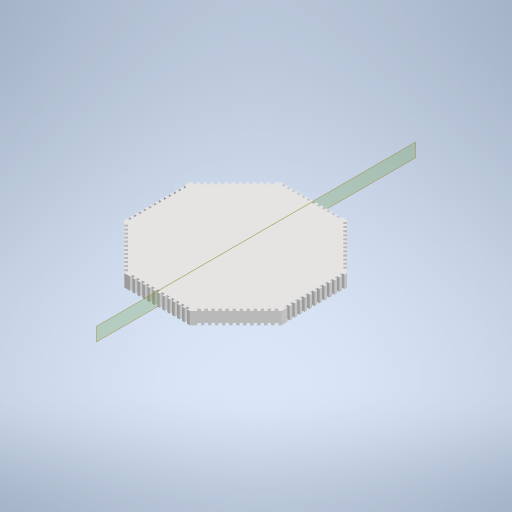
# Autodesk Inventor part: pla
Saved by Autodesk Inventor 2023 (Build 270158000, 158)
## iProperties
Created: 2023-04-19
Part Number: pla
Material: 일반
Document SubType Name: Modeling
Designer: didtk
Density: 1 g/cm^3
Appearance: 기본값
Author: didtk
Autodesk Inventor part; units mm, degrees
(part 1 of 2)
ref_plane "YZ Plane" through (0, 0, 0) normal (1, 0, 0) x (0, 1, 0)
ref_plane "XZ Plane" through (0, 0, 0) normal (0, 1, 0) x (-1, 0, 0)
ref_plane "XY Plane" through (0, 0, 0) normal (0, 0, 1) x (1, 0, 0)
sketch "스케치1" plane through (0, 0, 0) normal (0, 1, 0) x (-1, 0, 0)
  line L0 (26.6174, 64.26) -> (27.3245, 63.5529)
  line L1 (27.3245, 63.5529) -> (26.6174, 62.8458)
  line L2 (27.3245, 62.1387) -> (26.6174, 62.8458)
  line L3 (28.0316, 62.8458) -> (27.3245, 62.1387)
  line L4 (28.0316, 62.8458) -> (28.7387, 62.1387)
  line L5 (28.7387, 62.1387) -> (28.0316, 61.4316)
  line L6 (28.7387, 60.7245) -> (28.0316, 61.4316)
  line L7 (29.4458, 61.4316) -> (28.7387, 60.7245)
  line L8 (29.4458, 61.4316) -> (30.1529, 60.7245)
  line L9 (30.1529, 60.7245) -> (29.4458, 60.0174)
  line L10 (30.1529, 59.3103) -> (29.4458, 60.0174)
  line L11 (30.86, 60.0174) -> (30.1529, 59.3103)
  line L12 (30.86, 60.0174) -> (31.5671, 59.3103)
  line L13 (31.5671, 59.3103) -> (30.86, 58.6032)
  line L14 (31.5671, 57.896) -> (30.86, 58.6032)
  line L15 (32.2742, 58.6032) -> (31.5671, 57.896)
  line L16 (32.2742, 58.6032) -> (32.9813, 57.896)
  line L17 (32.9813, 57.896) -> (32.2742, 57.1889)
  line L18 (32.9813, 56.4818) -> (32.2742, 57.1889)
  line L19 (33.6884, 57.1889) -> (32.9813, 56.4818)
  line L20 (33.6884, 57.1889) -> (34.3955, 56.4818)
  line L21 (34.3955, 56.4818) -> (33.6884, 55.7747)
  line L22 (34.3955, 55.0676) -> (33.6884, 55.7747)
  line L23 (35.1026, 55.7747) -> (34.3955, 55.0676)
  line L24 (35.1026, 55.7747) -> (35.8098, 55.0676)
  line L25 (35.8098, 55.0676) -> (35.1026, 54.3605)
  line L26 (35.8098, 53.6534) -> (35.1026, 54.3605)
  line L27 (36.5169, 54.3605) -> (35.8098, 53.6534)
  line L28 (36.5169, 54.3605) -> (37.224, 53.6534)
  line L29 (37.224, 53.6534) -> (36.5169, 52.9463)
  line L30 (37.224, 52.2392) -> (36.5169, 52.9463)
  line L31 (37.9311, 52.9463) -> (37.224, 52.2392)
  line L32 (37.9311, 52.9463) -> (38.6382, 52.2392)
  line L33 (38.6382, 52.2392) -> (37.9311, 51.5321)
  line L34 (38.6382, 50.825) -> (37.9311, 51.5321)
  line L35 (39.3453, 51.5321) -> (38.6382, 50.825)
  line L36 (39.3453, 51.5321) -> (40.0524, 50.825)
  line L37 (40.0524, 50.825) -> (39.3453, 50.1179)
  line L38 (40.0524, 49.4108) -> (39.3453, 50.1179)
  line L39 (40.7595, 50.1179) -> (40.0524, 49.4108)
  line L40 (40.7595, 50.1179) -> (41.4666, 49.4108)
  line L41 (41.4666, 49.4108) -> (40.7595, 48.7037)
  line L42 (41.4666, 47.9965) -> (40.7595, 48.7037)
  line L43 (42.1737, 48.7037) -> (41.4666, 47.9965)
  line L44 (42.1737, 48.7037) -> (42.8808, 47.9965)
  line L45 (42.8808, 47.9965) -> (42.1737, 47.2894)
  line L46 (42.8808, 46.5823) -> (42.1737, 47.2894)
  line L47 (43.5879, 47.2894) -> (42.8808, 46.5823)
  line L48 (43.5879, 47.2894) -> (45.1681, 45.7092)
  line L49 (45.1681, 45.7092) -> (45.1681, 44.7092)
  line L50 (45.1681, 44.7092) -> (44.1681, 44.7092)
  line L51 (44.1681, 43.7092) -> (44.1681, 44.7092)
  line L52 (45.1681, 43.7092) -> (44.1681, 43.7092)
  line L53 (45.1681, 43.7092) -> (45.1681, 42.7092)
  line L54 (45.1681, 42.7092) -> (44.1681, 42.7092)
  line L55 (44.1681, 41.7092) -> (44.1681, 42.7092)
  line L56 (45.1681, 41.7092) -> (44.1681, 41.7092)
  line L57 (45.1681, 41.7092) -> (45.1681, 40.7092)
  line L58 (45.1681, 40.7092) -> (44.1681, 40.7092)
  line L59 (44.1681, 39.7092) -> (44.1681, 40.7092)
  line L60 (45.1681, 39.7092) -> (44.1681, 39.7092)
  line L61 (45.1681, 39.7092) -> (45.1681, 38.7092)
  line L62 (45.1681, 38.7092) -> (44.1681, 38.7092)
  line L63 (44.1681, 37.7092) -> (44.1681, 38.7092)
  line L64 (45.1681, 37.7092) -> (44.1681, 37.7092)
  line L65 (45.1681, 37.7092) -> (45.1681, 36.7092)
  line L66 (45.1681, 36.7092) -> (44.1681, 36.7092)
  line L67 (44.1681, 35.7092) -> (44.1681, 36.7092)
  line L68 (45.1681, 35.7092) -> (44.1681, 35.7092)
  line L69 (45.1681, 35.7092) -> (45.1681, 34.7092)
  line L70 (45.1681, 34.7092) -> (44.1681, 34.7092)
  line L71 (44.1681, 33.7092) -> (44.1681, 34.7092)
  line L72 (45.1681, 33.7092) -> (44.1681, 33.7092)
  line L73 (45.1681, 33.7092) -> (45.1681, 32.7092)
  line L74 (45.1681, 32.7092) -> (44.1681, 32.7092)
  line L75 (44.1681, 31.7092) -> (44.1681, 32.7092)
  line L76 (45.1681, 31.7092) -> (44.1681, 31.7092)
  line L77 (45.1681, 31.7092) -> (45.1681, 30.7092)
  line L78 (45.1681, 30.7092) -> (44.1681, 30.7092)
  line L79 (44.1681, 29.7092) -> (44.1681, 30.7092)
  line L80 (45.1681, 29.7092) -> (44.1681, 29.7092)
  line L81 (45.1681, 29.7092) -> (45.1681, 28.7092)
  line L82 (45.1681, 28.7092) -> (44.1681, 28.7092)
  line L83 (44.1681, 27.7092) -> (44.1681, 28.7092)
  line L84 (45.1681, 27.7092) -> (44.1681, 27.7092)
  line L85 (45.1681, 27.7092) -> (45.1681, 26.7092)
  line L86 (45.1681, 26.7092) -> (44.1681, 26.7092)
  line L87 (44.1681, 25.7092) -> (44.1681, 26.7092)
  line L88 (45.1681, 25.7092) -> (44.1681, 25.7092)
  line L89 (45.1681, 25.7092) -> (45.1681, 24.7092)
  line L90 (45.1681, 24.7092) -> (44.1681, 24.7092)
  line L91 (44.1681, 23.7092) -> (44.1681, 24.7092)
  line L92 (45.1681, 23.7092) -> (44.1681, 23.7092)
  line L93 (45.1681, 23.7092) -> (45.1681, 22.7092)
  line L94 (45.1681, 22.7092) -> (44.1681, 22.7092)
  line L95 (44.1681, 21.7092) -> (44.1681, 22.7092)
  line L96 (45.1681, 21.7092) -> (44.1681, 21.7092)
  line L97 (45.1681, 21.7092) -> (45.1681, 19.4745)
  line L98 (45.1681, 19.4745) -> (44.461, 18.7674)
  line L99 (44.461, 18.7674) -> (43.7539, 19.4745)
  line L100 (43.0468, 18.7674) -> (43.7539, 19.4745)
  line L101 (43.7539, 18.0603) -> (43.0468, 18.7674)
  line L102 (43.7539, 18.0603) -> (43.0468, 17.3532)
  line L103 (43.0468, 17.3532) -> (42.3397, 18.0603)
  line L104 (41.6326, 17.3532) -> (42.3397, 18.0603)
  line L105 (42.3397, 16.6461) -> (41.6326, 17.3532)
  line L106 (42.3397, 16.6461) -> (41.6326, 15.939)
  line L107 (41.6326, 15.939) -> (40.9255, 16.6461)
  line L108 (40.2184, 15.939) -> (40.9255, 16.6461)
  line L109 (40.9255, 15.2319) -> (40.2184, 15.939)
  line L110 (40.9255, 15.2319) -> (40.2184, 14.5248)
  line L111 (40.2184, 14.5248) -> (39.5113, 15.2319)
  line L112 (38.8042, 14.5248) -> (39.5113, 15.2319)
  line L113 (39.5113, 13.8177) -> (38.8042, 14.5248)
  line L114 (39.5113, 13.8177) -> (38.8042, 13.1106)
  line L115 (38.8042, 13.1106) -> (38.0971, 13.8177)
  line L116 (37.3899, 13.1106) -> (38.0971, 13.8177)
  line L117 (38.0971, 12.4034) -> (37.3899, 13.1106)
  line L118 (38.0971, 12.4034) -> (37.3899, 11.6963)
  line L119 (37.3899, 11.6963) -> (36.6828, 12.4034)
  line L120 (35.9757, 11.6963) -> (36.6828, 12.4034)
  line L121 (36.6828, 10.9892) -> (35.9757, 11.6963)
  line L122 (36.6828, 10.9892) -> (35.9757, 10.2821)
  line L123 (35.9757, 10.2821) -> (35.2686, 10.9892)
  line L124 (34.5615, 10.2821) -> (35.2686, 10.9892)
  line L125 (35.2686, 9.575) -> (34.5615, 10.2821)
  line L126 (35.2686, 9.575) -> (34.5615, 8.8679)
  line L127 (34.5615, 8.8679) -> (33.8544, 9.575)
  line L128 (33.1473, 8.8679) -> (33.8544, 9.575)
  line L129 (33.8544, 8.1608) -> (33.1473, 8.8679)
  line L130 (33.8544, 8.1608) -> (33.1473, 7.4537)
  line L131 (33.1473, 7.4537) -> (32.4402, 8.1608)
  line L132 (31.7331, 7.4537) -> (32.4402, 8.1608)
  line L133 (32.4402, 6.7466) -> (31.7331, 7.4537)
  line L134 (32.4402, 6.7466) -> (31.7331, 6.0395)
  line L135 (31.7331, 6.0395) -> (31.026, 6.7466)
  line L136 (30.3189, 6.0395) -> (31.026, 6.7466)
  line L137 (31.026, 5.3324) -> (30.3189, 6.0395)
  line L138 (31.026, 5.3324) -> (30.3189, 4.6253)
  line L139 (30.3189, 4.6253) -> (29.6118, 5.3324)
  line L140 (28.9047, 4.6253) -> (29.6118, 5.3324)
  line L141 (29.6118, 3.9182) -> (28.9047, 4.6253)
  line L142 (29.6118, 3.9182) -> (28.9047, 3.2111)
  line L143 (28.9047, 3.2111) -> (28.1976, 3.9182)
  line L144 (27.4905, 3.2111) -> (28.1976, 3.9182)
  line L145 (28.1976, 2.504) -> (27.4905, 3.2111)
  line L146 (28.1976, 2.504) -> (26.6174, 0.9238)
  line L147 (26.6174, 0.9238) -> (25.6174, 0.9238)
  line L148 (25.6174, 0.9238) -> (25.6174, 1.9238)
  line L149 (24.6174, 1.9238) -> (25.6174, 1.9238)
  line L150 (24.6174, 0.9238) -> (24.6174, 1.9238)
  line L151 (24.6174, 0.9238) -> (23.6174, 0.9238)
  line L152 (23.6174, 0.9238) -> (23.6174, 1.9238)
  line L153 (22.6174, 1.9238) -> (23.6174, 1.9238)
  line L154 (22.6174, 0.9238) -> (22.6174, 1.9238)
  line L155 (22.6174, 0.9238) -> (21.6174, 0.9238)
  line L156 (21.6174, 0.9238) -> (21.6174, 1.9238)
  line L157 (20.6174, 1.9238) -> (21.6174, 1.9238)
  line L158 (20.6174, 0.9238) -> (20.6174, 1.9238)
  line L159 (20.6174, 0.9238) -> (19.6174, 0.9238)
  line L160 (19.6174, 0.9238) -> (19.6174, 1.9238)
  line L161 (18.6174, 1.9238) -> (19.6174, 1.9238)
  line L162 (18.6174, 0.9238) -> (18.6174, 1.9238)
  line L163 (18.6174, 0.9238) -> (17.6174, 0.9238)
  line L164 (17.6174, 0.9238) -> (17.6174, 1.9238)
  line L165 (16.6174, 1.9238) -> (17.6174, 1.9238)
  line L166 (16.6174, 0.9238) -> (16.6174, 1.9238)
  line L167 (16.6174, 0.9238) -> (15.6174, 0.9238)
  line L168 (15.6174, 0.9238) -> (15.6174, 1.9238)
  line L169 (14.6174, 1.9238) -> (15.6174, 1.9238)
  line L170 (14.6174, 0.9238) -> (14.6174, 1.9238)
  line L171 (14.6174, 0.9238) -> (13.6174, 0.9238)
  line L172 (13.6174, 0.9238) -> (13.6174, 1.9238)
  line L173 (12.6174, 1.9238) -> (13.6174, 1.9238)
  line L174 (12.6174, 0.9238) -> (12.6174, 1.9238)
  line L175 (12.6174, 0.9238) -> (11.6174, 0.9238)
  line L176 (11.6174, 0.9238) -> (11.6174, 1.9238)
  line L177 (10.6174, 1.9238) -> (11.6174, 1.9238)
  line L178 (10.6174, 0.9238) -> (10.6174, 1.9238)
  line L179 (10.6174, 0.9238) -> (9.6174, 0.9238)
  line L180 (9.6174, 0.9238) -> (9.6174, 1.9238)
  line L181 (8.6174, 1.9238) -> (9.6174, 1.9238)
  line L182 (8.6174, 0.9238) -> (8.6174, 1.9238)
  line L183 (8.6174, 0.9238) -> (7.6174, 0.9238)
  line L184 (7.6174, 0.9238) -> (7.6174, 1.9238)
  line L185 (6.6174, 1.9238) -> (7.6174, 1.9238)
  line L186 (6.6174, 0.9238) -> (6.6174, 1.9238)
  line L187 (6.6174, 0.9238) -> (5.6174, 0.9238)
  line L188 (5.6174, 0.9238) -> (5.6174, 1.9238)
  line L189 (4.6174, 1.9238) -> (5.6174, 1.9238)
  line L190 (4.6174, 0.9238) -> (4.6174, 1.9238)
  line L191 (4.6174, 0.9238) -> (3.6174, 0.9238)
  line L192 (3.6174, 0.9238) -> (3.6174, 1.9238)
  line L193 (2.6174, 1.9238) -> (3.6174, 1.9238)
  line L194 (2.6174, 0.9238) -> (2.6174, 1.9238)
  line L195 (2.6174, 0.9238) -> (0.3826, 0.9238)
  line L196 (0.3826, 0.9238) -> (-0.3245, 1.6309)
  line L197 (-0.3245, 1.6309) -> (0.3826, 2.338)
  line L198 (-0.3245, 3.0451) -> (0.3826, 2.338)
  line L199 (-1.0316, 2.338) -> (-0.3245, 3.0451)
  line L200 (-1.0316, 2.338) -> (-1.7387, 3.0451)
  line L201 (-1.7387, 3.0451) -> (-1.0316, 3.7522)
  line L202 (-1.7387, 4.4593) -> (-1.0316, 3.7522)
  line L203 (-2.4458, 3.7522) -> (-1.7387, 4.4593)
  line L204 (-2.4458, 3.7522) -> (-3.1529, 4.4593)
  line L205 (-3.1529, 4.4593) -> (-2.4458, 5.1664)
  line L206 (-3.1529, 5.8735) -> (-2.4458, 5.1664)
  line L207 (-3.86, 5.1664) -> (-3.1529, 5.8735)
  line L208 (-3.86, 5.1664) -> (-4.5671, 5.8735)
  line L209 (-4.5671, 5.8735) -> (-3.86, 6.5806)
  line L210 (-4.5671, 7.2877) -> (-3.86, 6.5806)
  line L211 (-5.2742, 6.5806) -> (-4.5671, 7.2877)
  line L212 (-5.2742, 6.5806) -> (-5.9813, 7.2877)
  line L213 (-5.9813, 7.2877) -> (-5.2742, 7.9948)
  line L214 (-5.9813, 8.7019) -> (-5.2742, 7.9948)
  line L215 (-6.6884, 7.9948) -> (-5.9813, 8.7019)
  line L216 (-6.6884, 7.9948) -> (-7.3955, 8.7019)
  line L217 (-7.3955, 8.7019) -> (-6.6884, 9.409)
  line L218 (-7.3955, 10.1161) -> (-6.6884, 9.409)
  line L219 (-8.1026, 9.409) -> (-7.3955, 10.1161)
  line L220 (-8.1026, 9.409) -> (-8.8098, 10.1161)
  line L221 (-8.8098, 10.1161) -> (-8.1026, 10.8233)
  line L222 (-8.8098, 11.5304) -> (-8.1026, 10.8233)
  line L223 (-9.5169, 10.8233) -> (-8.8098, 11.5304)
  line L224 (-9.5169, 10.8233) -> (-10.224, 11.5304)
  line L225 (-10.224, 11.5304) -> (-9.5169, 12.2375)
  line L226 (-10.224, 12.9446) -> (-9.5169, 12.2375)
  line L227 (-10.9311, 12.2375) -> (-10.224, 12.9446)
  line L228 (-10.9311, 12.2375) -> (-11.6382, 12.9446)
  line L229 (-11.6382, 12.9446) -> (-10.9311, 13.6517)
  line L230 (-11.6382, 14.3588) -> (-10.9311, 13.6517)
  line L231 (-12.3453, 13.6517) -> (-11.6382, 14.3588)
  line L232 (-12.3453, 13.6517) -> (-13.0524, 14.3588)
  line L233 (-13.0524, 14.3588) -> (-12.3453, 15.0659)
  line L234 (-13.0524, 15.773) -> (-12.3453, 15.0659)
  line L235 (-13.7595, 15.0659) -> (-13.0524, 15.773)
  line L236 (-13.7595, 15.0659) -> (-14.4666, 15.773)
  line L237 (-14.4666, 15.773) -> (-13.7595, 16.4801)
  line L238 (-14.4666, 17.1872) -> (-13.7595, 16.4801)
  line L239 (-15.1737, 16.4801) -> (-14.4666, 17.1872)
  line L240 (-15.1737, 16.4801) -> (-15.8808, 17.1872)
  line L241 (-15.8808, 17.1872) -> (-15.1737, 17.8943)
  line L242 (-15.8808, 18.6014) -> (-15.1737, 17.8943)
  line L243 (-16.5879, 17.8943) -> (-15.8808, 18.6014)
  line L244 (-16.5879, 17.8943) -> (-18.1681, 19.4745)
  line L245 (-18.1681, 19.4745) -> (-18.1681, 20.4745)
  line L246 (-18.1681, 20.4745) -> (-17.1681, 20.4745)
  line L247 (-17.1681, 21.4745) -> (-17.1681, 20.4745)
  line L248 (-18.1681, 21.4745) -> (-17.1681, 21.4745)
  line L249 (-18.1681, 21.4745) -> (-18.1681, 22.4745)
  line L250 (-18.1681, 22.4745) -> (-17.1681, 22.4745)
  line L251 (-17.1681, 23.4745) -> (-17.1681, 22.4745)
  line L252 (-18.1681, 23.4745) -> (-17.1681, 23.4745)
  line L253 (-18.1681, 23.4745) -> (-18.1681, 24.4745)
  line L254 (-18.1681, 24.4745) -> (-17.1681, 24.4745)
  line L255 (-17.1681, 25.4745) -> (-17.1681, 24.4745)
  line L256 (-18.1681, 25.4745) -> (-17.1681, 25.4745)
  line L257 (-18.1681, 25.4745) -> (-18.1681, 26.4745)
  line L258 (-18.1681, 26.4745) -> (-17.1681, 26.4745)
  line L259 (-17.1681, 27.4745) -> (-17.1681, 26.4745)
  line L260 (-18.1681, 27.4745) -> (-17.1681, 27.4745)
  line L261 (-18.1681, 27.4745) -> (-18.1681, 28.4745)
  line L262 (-18.1681, 28.4745) -> (-17.1681, 28.4745)
  line L263 (-17.1681, 29.4745) -> (-17.1681, 28.4745)
  line L264 (-18.1681, 29.4745) -> (-17.1681, 29.4745)
  line L265 (-18.1681, 29.4745) -> (-18.1681, 30.4745)
  line L266 (-18.1681, 30.4745) -> (-17.1681, 30.4745)
  line L267 (-17.1681, 31.4745) -> (-17.1681, 30.4745)
  line L268 (-18.1681, 31.4745) -> (-17.1681, 31.4745)
  line L269 (-18.1681, 31.4745) -> (-18.1681, 32.4745)
  line L270 (-18.1681, 32.4745) -> (-17.1681, 32.4745)
  line L271 (-17.1681, 33.4745) -> (-17.1681, 32.4745)
  line L272 (-18.1681, 33.4745) -> (-17.1681, 33.4745)
  line L273 (-18.1681, 33.4745) -> (-18.1681, 34.4745)
  line L274 (-18.1681, 34.4745) -> (-17.1681, 34.4745)
  line L275 (-17.1681, 35.4745) -> (-17.1681, 34.4745)
  line L276 (-18.1681, 35.4745) -> (-17.1681, 35.4745)
  line L277 (-18.1681, 35.4745) -> (-18.1681, 36.4745)
  line L278 (-18.1681, 36.4745) -> (-17.1681, 36.4745)
  line L279 (-17.1681, 37.4745) -> (-17.1681, 36.4745)
  line L280 (-18.1681, 37.4745) -> (-17.1681, 37.4745)
  line L281 (-18.1681, 37.4745) -> (-18.1681, 38.4745)
  line L282 (-18.1681, 38.4745) -> (-17.1681, 38.4745)
  line L283 (-17.1681, 39.4745) -> (-17.1681, 38.4745)
  line L284 (-18.1681, 39.4745) -> (-17.1681, 39.4745)
  line L285 (-18.1681, 39.4745) -> (-18.1681, 40.4745)
  line L286 (-18.1681, 40.4745) -> (-17.1681, 40.4745)
  line L287 (-17.1681, 41.4745) -> (-17.1681, 40.4745)
  line L288 (-18.1681, 41.4745) -> (-17.1681, 41.4745)
  line L289 (-18.1681, 41.4745) -> (-18.1681, 42.4745)
  line L290 (-18.1681, 42.4745) -> (-17.1681, 42.4745)
  line L291 (-17.1681, 43.4745) -> (-17.1681, 42.4745)
  line L292 (-18.1681, 43.4745) -> (-17.1681, 43.4745)
  line L293 (-18.1681, 43.4745) -> (-18.1681, 45.7092)
  line L294 (-18.1681, 45.7092) -> (-17.461, 46.4164)
  line L295 (-17.461, 46.4164) -> (-16.7539, 45.7092)
  line L296 (-16.0468, 46.4164) -> (-16.7539, 45.7092)
  line L297 (-16.7539, 47.1235) -> (-16.0468, 46.4164)
  line L298 (-16.7539, 47.1235) -> (-16.0468, 47.8306)
  line L299 (-16.0468, 47.8306) -> (-15.3397, 47.1235)
  line L300 (-14.6326, 47.8306) -> (-15.3397, 47.1235)
  line L301 (-15.3397, 48.5377) -> (-14.6326, 47.8306)
  line L302 (-15.3397, 48.5377) -> (-14.6326, 49.2448)
  line L303 (-14.6326, 49.2448) -> (-13.9255, 48.5377)
  line L304 (-13.2184, 49.2448) -> (-13.9255, 48.5377)
  line L305 (-13.9255, 49.9519) -> (-13.2184, 49.2448)
  line L306 (-13.9255, 49.9519) -> (-13.2184, 50.659)
  line L307 (-13.2184, 50.659) -> (-12.5113, 49.9519)
  line L308 (-11.8042, 50.659) -> (-12.5113, 49.9519)
  line L309 (-12.5113, 51.3661) -> (-11.8042, 50.659)
  line L310 (-12.5113, 51.3661) -> (-11.8042, 52.0732)
  line L311 (-11.8042, 52.0732) -> (-11.0971, 51.3661)
  line L312 (-10.3899, 52.0732) -> (-11.0971, 51.3661)
  line L313 (-11.0971, 52.7803) -> (-10.3899, 52.0732)
  line L314 (-11.0971, 52.7803) -> (-10.3899, 53.4874)
  line L315 (-10.3899, 53.4874) -> (-9.6828, 52.7803)
  line L316 (-8.9757, 53.4874) -> (-9.6828, 52.7803)
  line L317 (-9.6828, 54.1945) -> (-8.9757, 53.4874)
  line L318 (-9.6828, 54.1945) -> (-8.9757, 54.9016)
  line L319 (-8.9757, 54.9016) -> (-8.2686, 54.1945)
  line L320 (-7.5615, 54.9016) -> (-8.2686, 54.1945)
  line L321 (-8.2686, 55.6087) -> (-7.5615, 54.9016)
  line L322 (-8.2686, 55.6087) -> (-7.5615, 56.3159)
  line L323 (-7.5615, 56.3159) -> (-6.8544, 55.6087)
  line L324 (-6.1473, 56.3159) -> (-6.8544, 55.6087)
  line L325 (-6.8544, 57.023) -> (-6.1473, 56.3159)
  line L326 (-6.8544, 57.023) -> (-6.1473, 57.7301)
  line L327 (-6.1473, 57.7301) -> (-5.4402, 57.023)
  line L328 (-4.7331, 57.7301) -> (-5.4402, 57.023)
  line L329 (-5.4402, 58.4372) -> (-4.7331, 57.7301)
  line L330 (-5.4402, 58.4372) -> (-4.7331, 59.1443)
  line L331 (-4.7331, 59.1443) -> (-4.026, 58.4372)
  line L332 (-3.3189, 59.1443) -> (-4.026, 58.4372)
  line L333 (-4.026, 59.8514) -> (-3.3189, 59.1443)
  line L334 (-4.026, 59.8514) -> (-3.3189, 60.5585)
  line L335 (-3.3189, 60.5585) -> (-2.6118, 59.8514)
  line L336 (-1.9047, 60.5585) -> (-2.6118, 59.8514)
  line L337 (-2.6118, 61.2656) -> (-1.9047, 60.5585)
  line L338 (-2.6118, 61.2656) -> (-1.9047, 61.9727)
  line L339 (-1.9047, 61.9727) -> (-1.1976, 61.2656)
  line L340 (-0.4905, 61.9727) -> (-1.1976, 61.2656)
  line L341 (-1.1976, 62.6798) -> (-0.4905, 61.9727)
  line L342 (-1.1976, 62.6798) -> (0.3826, 64.26)
  line L343 (0.3826, 64.26) -> (1.3826, 64.26)
  line L344 (1.3826, 64.26) -> (1.3826, 63.26)
  line L345 (2.3826, 63.26) -> (1.3826, 63.26)
  line L346 (2.3826, 64.26) -> (2.3826, 63.26)
  line L347 (2.3826, 64.26) -> (3.3826, 64.26)
  line L348 (3.3826, 64.26) -> (3.3826, 63.26)
  line L349 (4.3826, 63.26) -> (3.3826, 63.26)
  line L350 (4.3826, 64.26) -> (4.3826, 63.26)
  line L351 (4.3826, 64.26) -> (5.3826, 64.26)
  line L352 (5.3826, 64.26) -> (5.3826, 63.26)
  line L353 (6.3826, 63.26) -> (5.3826, 63.26)
  line L354 (6.3826, 64.26) -> (6.3826, 63.26)
  line L355 (6.3826, 64.26) -> (7.3826, 64.26)
  line L356 (7.3826, 64.26) -> (7.3826, 63.26)
  line L357 (8.3826, 63.26) -> (7.3826, 63.26)
  line L358 (8.3826, 64.26) -> (8.3826, 63.26)
  line L359 (8.3826, 64.26) -> (9.3826, 64.26)
  line L360 (9.3826, 64.26) -> (9.3826, 63.26)
  line L361 (10.3826, 63.26) -> (9.3826, 63.26)
  line L362 (10.3826, 64.26) -> (10.3826, 63.26)
  line L363 (10.3826, 64.26) -> (11.3826, 64.26)
  line L364 (11.3826, 64.26) -> (11.3826, 63.26)
  line L365 (12.3826, 63.26) -> (11.3826, 63.26)
  line L366 (12.3826, 64.26) -> (12.3826, 63.26)
  line L367 (12.3826, 64.26) -> (13.3826, 64.26)
  line L368 (13.3826, 64.26) -> (13.3826, 63.26)
  line L369 (14.3826, 63.26) -> (13.3826, 63.26)
  line L370 (14.3826, 64.26) -> (14.3826, 63.26)
  line L371 (14.3826, 64.26) -> (15.3826, 64.26)
  line L372 (15.3826, 64.26) -> (15.3826, 63.26)
  line L373 (16.3826, 63.26) -> (15.3826, 63.26)
  line L374 (16.3826, 64.26) -> (16.3826, 63.26)
  line L375 (16.3826, 64.26) -> (17.3826, 64.26)
  line L376 (17.3826, 64.26) -> (17.3826, 63.26)
  line L377 (18.3826, 63.26) -> (17.3826, 63.26)
  line L378 (18.3826, 64.26) -> (18.3826, 63.26)
  line L379 (18.3826, 64.26) -> (19.3826, 64.26)
  line L380 (19.3826, 64.26) -> (19.3826, 63.26)
  line L381 (20.3826, 63.26) -> (19.3826, 63.26)
  line L382 (20.3826, 64.26) -> (20.3826, 63.26)
  line L383 (20.3826, 64.26) -> (21.3826, 64.26)
  line L384 (21.3826, 64.26) -> (21.3826, 63.26)
  line L385 (22.3826, 63.26) -> (21.3826, 63.26)
  line L386 (22.3826, 64.26) -> (22.3826, 63.26)
  line L387 (22.3826, 64.26) -> (23.3826, 64.26)
  line L388 (23.3826, 64.26) -> (23.3826, 63.26)
  line L389 (24.3826, 63.26) -> (23.3826, 63.26)
  line L390 (24.3826, 64.26) -> (24.3826, 63.26)
  line L391 (24.3826, 64.26) -> (26.6174, 64.26)
  line L392 (37.6421, 22.5919) -> (23.5, 8.4497)
  line L393 (23.5, 8.4497) -> (3.5, 8.4497)
  line L394 (3.5, 8.4497) -> (-10.6421, 22.5919)
  line L395 (-10.6421, 22.5919) -> (-10.6421, 42.5919)
  line L396 (-10.6421, 42.5919) -> (3.5, 56.734)
  line L397 (3.5, 56.734) -> (23.5, 56.734)
  line L398 (23.5, 56.734) -> (37.6421, 42.5919)
  line L399 (37.6421, 42.5919) -> (37.6421, 22.5919)
  point P0 (0, 0)
  point P1 (13.5, 32.5919)
  point P2 (13.5, 32.5919)
  dimension "d0" = 31.6681
  dimension "d1" = 31.6681
  dimension "d2" = 31.6681
  dimension "d3" = 31.6681
  dimension "d4" = 35.2772
  dimension "d5" = 20
  constraints: 800 end point, 1 coincident, 17 other
  measures "d0" distance from line of L371 point (13.5, 32.592)
  measures "d1" distance from line of L171 point (13.5, 32.592)
  measures "d2" distance from line of L73 point (13.5, 32.592)
  measures "d3" distance from line of L269 point (13.5, 32.592)
  measures "d4" distance of point (13.5, 32.592) point (0, 0)
  measures "d5" distance of L398.end L392.start
extrude "돌출1" add sketch "스케치1" along normal blind 5
sketch "스케치2" plane through (0, 0, 0) normal (0, 1, 0) x (-1, 0, 0)
  line L0 (29.4458, 60.0174) -> (30.1529, 60.7245) projected
  line L1 (30.1529, 60.7245) -> (29.4458, 61.4316) projected
  line L2 (29.4458, 61.4316) -> (28.7387, 60.7245) projected
  line L3 (28.7387, 60.7245) -> (28.0316, 61.4316) projected
  line L4 (28.0316, 61.4316) -> (28.7387, 62.1387) projected
  line L5 (28.7387, 62.1387) -> (28.0316, 62.8458) projected
  line L6 (28.0316, 62.8458) -> (27.3245, 62.1387) projected
  line L7 (27.3245, 62.1387) -> (26.6174, 62.8458) projected
  line L8 (26.6174, 62.8458) -> (27.3245, 63.5529) projected
  line L9 (27.3245, 63.5529) -> (26.6174, 64.26) projected
  line L10 (26.6174, 64.26) -> (24.3826, 64.26) projected
  line L11 (24.3826, 64.26) -> (24.3826, 63.26) projected
  line L12 (24.3826, 63.26) -> (23.3826, 63.26) projected
  line L13 (23.3826, 63.26) -> (23.3826, 64.26) projected
  line L14 (23.3826, 64.26) -> (22.3826, 64.26) projected
  line L15 (22.3826, 64.26) -> (22.3826, 63.26) projected
  line L16 (22.3826, 63.26) -> (21.3826, 63.26) projected
  line L17 (21.3826, 63.26) -> (21.3826, 64.26) projected
  line L18 (21.3826, 64.26) -> (20.3826, 64.26) projected
  line L19 (20.3826, 64.26) -> (20.3826, 63.26) projected
  line L20 (20.3826, 63.26) -> (19.3826, 63.26) projected
  line L21 (19.3826, 63.26) -> (19.3826, 64.26) projected
  line L22 (19.3826, 64.26) -> (18.3826, 64.26) projected
  line L23 (18.3826, 64.26) -> (18.3826, 63.26) projected
  line L24 (18.3826, 63.26) -> (17.3826, 63.26) projected
  line L25 (17.3826, 63.26) -> (17.3826, 64.26) projected
  line L26 (17.3826, 64.26) -> (16.3826, 64.26) projected
  line L27 (16.3826, 64.26) -> (16.3826, 63.26) projected
  line L28 (16.3826, 63.26) -> (15.3826, 63.26) projected
  line L29 (15.3826, 63.26) -> (15.3826, 64.26) projected
  line L30 (15.3826, 64.26) -> (14.3826, 64.26) projected
  line L31 (14.3826, 64.26) -> (14.3826, 63.26) projected
  line L32 (14.3826, 63.26) -> (13.3826, 63.26) projected
  line L33 (13.3826, 63.26) -> (13.3826, 64.26) projected
  line L34 (13.3826, 64.26) -> (12.3826, 64.26) projected
  line L35 (12.3826, 64.26) -> (12.3826, 63.26) projected
  line L36 (12.3826, 63.26) -> (11.3826, 63.26) projected
  line L37 (11.3826, 63.26) -> (11.3826, 64.26) projected
  line L38 (11.3826, 64.26) -> (10.3826, 64.26) projected
  line L39 (10.3826, 64.26) -> (10.3826, 63.26) projected
  line L40 (10.3826, 63.26) -> (9.3826, 63.26) projected
  line L41 (9.3826, 63.26) -> (9.3826, 64.26) projected
  line L42 (9.3826, 64.26) -> (8.3826, 64.26) projected
  line L43 (8.3826, 64.26) -> (8.3826, 63.26) projected
  line L44 (8.3826, 63.26) -> (7.3826, 63.26) projected
  line L45 (7.3826, 63.26) -> (7.3826, 64.26) projected
  line L46 (7.3826, 64.26) -> (6.3826, 64.26) projected
  line L47 (6.3826, 64.26) -> (6.3826, 63.26) projected
  line L48 (6.3826, 63.26) -> (5.3826, 63.26) projected
  line L49 (5.3826, 63.26) -> (5.3826, 64.26) projected
  line L50 (5.3826, 64.26) -> (4.3826, 64.26) projected
  line L51 (4.3826, 64.26) -> (4.3826, 63.26) projected
  line L52 (4.3826, 63.26) -> (3.3826, 63.26) projected
  line L53 (3.3826, 63.26) -> (3.3826, 64.26) projected
  line L54 (3.3826, 64.26) -> (2.3826, 64.26) projected
  line L55 (2.3826, 64.26) -> (2.3826, 63.26) projected
  line L56 (2.3826, 63.26) -> (1.3826, 63.26) projected
  line L57 (1.3826, 63.26) -> (1.3826, 64.26) projected
  line L58 (1.3826, 64.26) -> (0.3826, 64.26) projected
  line L59 (0.3826, 64.26) -> (-1.1976, 62.6798) projected
  line L60 (-1.1976, 62.6798) -> (-0.4905, 61.9727) projected
  line L61 (-0.4905, 61.9727) -> (-1.1976, 61.2656) projected
  line L62 (-1.1976, 61.2656) -> (-1.9047, 61.9727) projected
  line L63 (-1.9047, 61.9727) -> (-2.6118, 61.2656) projected
  line L64 (-2.6118, 61.2656) -> (-1.9047, 60.5585) projected
  line L65 (-1.9047, 60.5585) -> (-2.6118, 59.8514) projected
  line L66 (-2.6118, 59.8514) -> (-3.3189, 60.5585) projected
  line L67 (-3.3189, 60.5585) -> (-4.026, 59.8514) projected
  line L68 (-4.026, 59.8514) -> (-3.3189, 59.1443) projected
  line L69 (-3.3189, 59.1443) -> (-4.026, 58.4372) projected
  line L70 (-4.026, 58.4372) -> (-4.7331, 59.1443) projected
  line L71 (-4.7331, 59.1443) -> (-5.4402, 58.4372) projected
  line L72 (-5.4402, 58.4372) -> (-4.7331, 57.7301) projected
  line L73 (-4.7331, 57.7301) -> (-5.4402, 57.023) projected
  line L74 (-5.4402, 57.023) -> (-6.1473, 57.7301) projected
  line L75 (-6.1473, 57.7301) -> (-6.8544, 57.023) projected
  line L76 (-6.8544, 57.023) -> (-6.1473, 56.3159) projected
  line L77 (-6.1473, 56.3159) -> (-6.8544, 55.6087) projected
  line L78 (-6.8544, 55.6087) -> (-7.5615, 56.3159) projected
  line L79 (-7.5615, 56.3159) -> (-8.2686, 55.6087) projected
  line L80 (-8.2686, 55.6087) -> (-7.5615, 54.9016) projected
  line L81 (-7.5615, 54.9016) -> (-8.2686, 54.1945) projected
  line L82 (-8.2686, 54.1945) -> (-8.9757, 54.9016) projected
  line L83 (-8.9757, 54.9016) -> (-9.6828, 54.1945) projected
  line L84 (-9.6828, 54.1945) -> (-8.9757, 53.4874) projected
  line L85 (-8.9757, 53.4874) -> (-9.6828, 52.7803) projected
  line L86 (-9.6828, 52.7803) -> (-10.3899, 53.4874) projected
  line L87 (-10.3899, 53.4874) -> (-11.0971, 52.7803) projected
  line L88 (-11.0971, 52.7803) -> (-10.3899, 52.0732) projected
  line L89 (-10.3899, 52.0732) -> (-11.0971, 51.3661) projected
  line L90 (-11.0971, 51.3661) -> (-11.8042, 52.0732) projected
  line L91 (-11.8042, 52.0732) -> (-12.5113, 51.3661) projected
  line L92 (-12.5113, 51.3661) -> (-11.8042, 50.659) projected
  line L93 (-11.8042, 50.659) -> (-12.5113, 49.9519) projected
  line L94 (-12.5113, 49.9519) -> (-13.2184, 50.659) projected
  line L95 (-13.2184, 50.659) -> (-13.9255, 49.9519) projected
  line L96 (-13.9255, 49.9519) -> (-13.2184, 49.2448) projected
  line L97 (-13.2184, 49.2448) -> (-13.9255, 48.5377) projected
  line L98 (-13.9255, 48.5377) -> (-14.6326, 49.2448) projected
  line L99 (-14.6326, 49.2448) -> (-15.3397, 48.5377) projected
  line L100 (-15.3397, 48.5377) -> (-14.6326, 47.8306) projected
  line L101 (-14.6326, 47.8306) -> (-15.3397, 47.1235) projected
  line L102 (-15.3397, 47.1235) -> (-16.0468, 47.8306) projected
  line L103 (-16.0468, 47.8306) -> (-16.7539, 47.1235) projected
  line L104 (-16.7539, 47.1235) -> (-16.0468, 46.4164) projected
  line L105 (-16.0468, 46.4164) -> (-16.7539, 45.7092) projected
  line L106 (-16.7539, 45.7092) -> (-17.461, 46.4164) projected
  line L107 (-17.461, 46.4164) -> (-18.1681, 45.7092) projected
  line L108 (-18.1681, 45.7092) -> (-18.1681, 43.4745) projected
  line L109 (-18.1681, 43.4745) -> (-17.1681, 43.4745) projected
  line L110 (-17.1681, 43.4745) -> (-17.1681, 42.4745) projected
  line L111 (-17.1681, 42.4745) -> (-18.1681, 42.4745) projected
  line L112 (-18.1681, 42.4745) -> (-18.1681, 41.4745) projected
  line L113 (-18.1681, 41.4745) -> (-17.1681, 41.4745) projected
  line L114 (-17.1681, 41.4745) -> (-17.1681, 40.4745) projected
  line L115 (-17.1681, 40.4745) -> (-18.1681, 40.4745) projected
  line L116 (-18.1681, 40.4745) -> (-18.1681, 39.4745) projected
  line L117 (-18.1681, 39.4745) -> (-17.1681, 39.4745) projected
  line L118 (-17.1681, 39.4745) -> (-17.1681, 38.4745) projected
  line L119 (-17.1681, 38.4745) -> (-18.1681, 38.4745) projected
  line L120 (-18.1681, 38.4745) -> (-18.1681, 37.4745) projected
  line L121 (-18.1681, 37.4745) -> (-17.1681, 37.4745) projected
  line L122 (-17.1681, 37.4745) -> (-17.1681, 36.4745) projected
  line L123 (-17.1681, 36.4745) -> (-18.1681, 36.4745) projected
  line L124 (-18.1681, 36.4745) -> (-18.1681, 35.4745) projected
  line L125 (-18.1681, 35.4745) -> (-17.1681, 35.4745) projected
  line L126 (-17.1681, 35.4745) -> (-17.1681, 34.4745) projected
  line L127 (-17.1681, 34.4745) -> (-18.1681, 34.4745) projected
  line L128 (-18.1681, 34.4745) -> (-18.1681, 33.4745) projected
  line L129 (-18.1681, 33.4745) -> (-17.1681, 33.4745) projected
  line L130 (-17.1681, 33.4745) -> (-17.1681, 32.4745) projected
  line L131 (-17.1681, 32.4745) -> (-18.1681, 32.4745) projected
  line L132 (-18.1681, 32.4745) -> (-18.1681, 31.4745) projected
  line L133 (-18.1681, 31.4745) -> (-17.1681, 31.4745) projected
  line L134 (-17.1681, 31.4745) -> (-17.1681, 30.4745) projected
  line L135 (-17.1681, 30.4745) -> (-18.1681, 30.4745) projected
  line L136 (-18.1681, 30.4745) -> (-18.1681, 29.4745) projected
  line L137 (-18.1681, 29.4745) -> (-17.1681, 29.4745) projected
  line L138 (-17.1681, 29.4745) -> (-17.1681, 28.4745) projected
  line L139 (-17.1681, 28.4745) -> (-18.1681, 28.4745) projected
  line L140 (-18.1681, 28.4745) -> (-18.1681, 27.4745) projected
  line L141 (-18.1681, 27.4745) -> (-17.1681, 27.4745) projected
  line L142 (-17.1681, 27.4745) -> (-17.1681, 26.4745) projected
  line L143 (-17.1681, 26.4745) -> (-18.1681, 26.4745) projected
  line L144 (-18.1681, 26.4745) -> (-18.1681, 25.4745) projected
  line L145 (-18.1681, 25.4745) -> (-17.1681, 25.4745) projected
  line L146 (-17.1681, 25.4745) -> (-17.1681, 24.4745) projected
  line L147 (-17.1681, 24.4745) -> (-18.1681, 24.4745) projected
  line L148 (-18.1681, 24.4745) -> (-18.1681, 23.4745) projected
  line L149 (-18.1681, 23.4745) -> (-17.1681, 23.4745) projected
  line L150 (-17.1681, 23.4745) -> (-17.1681, 22.4745) projected
  line L151 (-17.1681, 22.4745) -> (-18.1681, 22.4745) projected
  line L152 (-18.1681, 22.4745) -> (-18.1681, 21.4745) projected
  line L153 (-18.1681, 21.4745) -> (-17.1681, 21.4745) projected
  line L154 (-17.1681, 21.4745) -> (-17.1681, 20.4745) projected
  line L155 (-17.1681, 20.4745) -> (-18.1681, 20.4745) projected
  line L156 (-18.1681, 20.4745) -> (-18.1681, 19.4745) projected
  line L157 (-18.1681, 19.4745) -> (-16.5879, 17.8943) projected
  line L158 (-16.5879, 17.8943) -> (-15.8808, 18.6014) projected
  line L159 (-15.8808, 18.6014) -> (-15.1737, 17.8943) projected
  line L160 (-15.1737, 17.8943) -> (-15.8808, 17.1872) projected
  line L161 (-15.8808, 17.1872) -> (-15.1737, 16.4801) projected
  line L162 (-15.1737, 16.4801) -> (-14.4666, 17.1872) projected
  line L163 (-14.4666, 17.1872) -> (-13.7595, 16.4801) projected
  line L164 (-13.7595, 16.4801) -> (-14.4666, 15.773) projected
  line L165 (-14.4666, 15.773) -> (-13.7595, 15.0659) projected
  line L166 (-13.7595, 15.0659) -> (-13.0524, 15.773) projected
  line L167 (-13.0524, 15.773) -> (-12.3453, 15.0659) projected
  line L168 (-12.3453, 15.0659) -> (-13.0524, 14.3588) projected
  line L169 (-13.0524, 14.3588) -> (-12.3453, 13.6517) projected
  line L170 (-12.3453, 13.6517) -> (-11.6382, 14.3588) projected
  line L171 (-11.6382, 14.3588) -> (-10.9311, 13.6517) projected
  line L172 (-10.9311, 13.6517) -> (-11.6382, 12.9446) projected
  line L173 (-11.6382, 12.9446) -> (-10.9311, 12.2375) projected
  line L174 (-10.9311, 12.2375) -> (-10.224, 12.9446) projected
  line L175 (-10.224, 12.9446) -> (-9.5169, 12.2375) projected
  line L176 (-9.5169, 12.2375) -> (-10.224, 11.5304) projected
  line L177 (-10.224, 11.5304) -> (-9.5169, 10.8233) projected
  line L178 (-9.5169, 10.8233) -> (-8.8098, 11.5304) projected
  line L179 (-8.8098, 11.5304) -> (-8.1026, 10.8233) projected
  line L180 (-8.1026, 10.8233) -> (-8.8098, 10.1161) projected
  line L181 (-8.8098, 10.1161) -> (-8.1026, 9.409) projected
  line L182 (-8.1026, 9.409) -> (-7.3955, 10.1161) projected
  line L183 (-7.3955, 10.1161) -> (-6.6884, 9.409) projected
  line L184 (-6.6884, 9.409) -> (-7.3955, 8.7019) projected
  line L185 (-7.3955, 8.7019) -> (-6.6884, 7.9948) projected
  line L186 (-6.6884, 7.9948) -> (-5.9813, 8.7019) projected
  line L187 (-5.9813, 8.7019) -> (-5.2742, 7.9948) projected
  line L188 (-5.2742, 7.9948) -> (-5.9813, 7.2877) projected
  line L189 (-5.9813, 7.2877) -> (-5.2742, 6.5806) projected
  line L190 (-5.2742, 6.5806) -> (-4.5671, 7.2877) projected
  line L191 (-4.5671, 7.2877) -> (-3.86, 6.5806) projected
  line L192 (-3.86, 6.5806) -> (-4.5671, 5.8735) projected
  line L193 (-4.5671, 5.8735) -> (-3.86, 5.1664) projected
  line L194 (-3.86, 5.1664) -> (-3.1529, 5.8735) projected
  line L195 (-3.1529, 5.8735) -> (-2.4458, 5.1664) projected
  line L196 (-2.4458, 5.1664) -> (-3.1529, 4.4593) projected
  line L197 (-3.1529, 4.4593) -> (-2.4458, 3.7522) projected
  line L198 (-2.4458, 3.7522) -> (-1.7387, 4.4593) projected
  line L199 (-1.7387, 4.4593) -> (-1.0316, 3.7522) projected
  line L200 (-1.0316, 3.7522) -> (-1.7387, 3.0451) projected
  line L201 (-1.7387, 3.0451) -> (-1.0316, 2.338) projected
  line L202 (-1.0316, 2.338) -> (-0.3245, 3.0451) projected
  line L203 (-0.3245, 3.0451) -> (0.3826, 2.338) projected
  line L204 (0.3826, 2.338) -> (-0.3245, 1.6309) projected
  line L205 (-0.3245, 1.6309) -> (0.3826, 0.9238) projected
  line L206 (0.3826, 0.9238) -> (2.6174, 0.9238) projected
  line L207 (2.6174, 0.9238) -> (2.6174, 1.9238) projected
  line L208 (2.6174, 1.9238) -> (3.6174, 1.9238) projected
  line L209 (3.6174, 1.9238) -> (3.6174, 0.9238) projected
  line L210 (3.6174, 0.9238) -> (4.6174, 0.9238) projected
  line L211 (4.6174, 0.9238) -> (4.6174, 1.9238) projected
  line L212 (4.6174, 1.9238) -> (5.6174, 1.9238) projected
  line L213 (5.6174, 1.9238) -> (5.6174, 0.9238) projected
  line L214 (5.6174, 0.9238) -> (6.6174, 0.9238) projected
  line L215 (6.6174, 0.9238) -> (6.6174, 1.9238) projected
  line L216 (6.6174, 1.9238) -> (7.6174, 1.9238) projected
  line L217 (7.6174, 1.9238) -> (7.6174, 0.9238) projected
  line L218 (7.6174, 0.9238) -> (8.6174, 0.9238) projected
  line L219 (8.6174, 0.9238) -> (8.6174, 1.9238) projected
  line L220 (8.6174, 1.9238) -> (9.6174, 1.9238) projected
  line L221 (9.6174, 1.9238) -> (9.6174, 0.9238) projected
  line L222 (9.6174, 0.9238) -> (10.6174, 0.9238) projected
  line L223 (10.6174, 0.9238) -> (10.6174, 1.9238) projected
  line L224 (10.6174, 1.9238) -> (11.6174, 1.9238) projected
  line L225 (11.6174, 1.9238) -> (11.6174, 0.9238) projected
  line L226 (11.6174, 0.9238) -> (12.6174, 0.9238) projected
  line L227 (12.6174, 0.9238) -> (12.6174, 1.9238) projected
  line L228 (12.6174, 1.9238) -> (13.6174, 1.9238) projected
  line L229 (13.6174, 1.9238) -> (13.6174, 0.9238) projected
  line L230 (13.6174, 0.9238) -> (14.6174, 0.9238) projected
  line L231 (14.6174, 0.9238) -> (14.6174, 1.9238) projected
  line L232 (14.6174, 1.9238) -> (15.6174, 1.9238) projected
  line L233 (15.6174, 1.9238) -> (15.6174, 0.9238) projected
  line L234 (15.6174, 0.9238) -> (16.6174, 0.9238) projected
  line L235 (16.6174, 0.9238) -> (16.6174, 1.9238) projected
  line L236 (16.6174, 1.9238) -> (17.6174, 1.9238) projected
  line L237 (17.6174, 1.9238) -> (17.6174, 0.9238) projected
  line L238 (17.6174, 0.9238) -> (18.6174, 0.9238) projected
  line L239 (18.6174, 0.9238) -> (18.6174, 1.9238) projected
  line L240 (18.6174, 1.9238) -> (19.6174, 1.9238) projected
  line L241 (19.6174, 1.9238) -> (19.6174, 0.9238) projected
  line L242 (19.6174, 0.9238) -> (20.6174, 0.9238) projected
  line L243 (20.6174, 0.9238) -> (20.6174, 1.9238) projected
  line L244 (20.6174, 1.9238) -> (21.6174, 1.9238) projected
  line L245 (21.6174, 1.9238) -> (21.6174, 0.9238) projected
  line L246 (21.6174, 0.9238) -> (22.6174, 0.9238) projected
  line L247 (22.6174, 0.9238) -> (22.6174, 1.9238) projected
  line L248 (22.6174, 1.9238) -> (23.6174, 1.9238) projected
  line L249 (23.6174, 1.9238) -> (23.6174, 0.9238) projected
  line L250 (23.6174, 0.9238) -> (24.6174, 0.9238) projected
  line L251 (24.6174, 0.9238) -> (24.6174, 1.9238) projected
  line L252 (24.6174, 1.9238) -> (25.6174, 1.9238) projected
  line L253 (25.6174, 1.9238) -> (25.6174, 0.9238) projected
  line L254 (25.6174, 0.9238) -> (26.6174, 0.9238) projected
  line L255 (26.6174, 0.9238) -> (28.1976, 2.504) projected
  line L256 (28.1976, 2.504) -> (27.4905, 3.2111) projected
  line L257 (27.4905, 3.2111) -> (28.1976, 3.9182) projected
  line L258 (28.1976, 3.9182) -> (28.9047, 3.2111) projected
  line L259 (28.9047, 3.2111) -> (29.6118, 3.9182) projected
  line L260 (29.6118, 3.9182) -> (28.9047, 4.6253) projected
  line L261 (28.9047, 4.6253) -> (29.6118, 5.3324) projected
  line L262 (29.6118, 5.3324) -> (30.3189, 4.6253) projected
  line L263 (30.3189, 4.6253) -> (31.026, 5.3324) projected
  line L264 (31.026, 5.3324) -> (30.3189, 6.0395) projected
  line L265 (30.3189, 6.0395) -> (31.026, 6.7466) projected
  line L266 (31.026, 6.7466) -> (31.7331, 6.0395) projected
  line L267 (31.7331, 6.0395) -> (32.4402, 6.7466) projected
  line L268 (32.4402, 6.7466) -> (31.7331, 7.4537) projected
  line L269 (31.7331, 7.4537) -> (32.4402, 8.1608) projected
  line L270 (32.4402, 8.1608) -> (33.1473, 7.4537) projected
  line L271 (33.1473, 7.4537) -> (33.8544, 8.1608) projected
  line L272 (33.8544, 8.1608) -> (33.1473, 8.8679) projected
  line L273 (33.1473, 8.8679) -> (33.8544, 9.575) projected
  line L274 (33.8544, 9.575) -> (34.5615, 8.8679) projected
  line L275 (34.5615, 8.8679) -> (35.2686, 9.575) projected
  line L276 (35.2686, 9.575) -> (34.5615, 10.2821) projected
  line L277 (34.5615, 10.2821) -> (35.2686, 10.9892) projected
  line L278 (35.2686, 10.9892) -> (35.9757, 10.2821) projected
  line L279 (35.9757, 10.2821) -> (36.6828, 10.9892) projected
  line L280 (36.6828, 10.9892) -> (35.9757, 11.6963) projected
  line L281 (35.9757, 11.6963) -> (36.6828, 12.4034) projected
  line L282 (36.6828, 12.4034) -> (37.3899, 11.6963) projected
  line L283 (37.3899, 11.6963) -> (38.0971, 12.4034) projected
  line L284 (38.0971, 12.4034) -> (37.3899, 13.1106) projected
  line L285 (37.3899, 13.1106) -> (38.0971, 13.8177) projected
  line L286 (38.0971, 13.8177) -> (38.8042, 13.1106) projected
  line L287 (38.8042, 13.1106) -> (39.5113, 13.8177) projected
  line L288 (39.5113, 13.8177) -> (38.8042, 14.5248) projected
  line L289 (38.8042, 14.5248) -> (39.5113, 15.2319) projected
  line L290 (39.5113, 15.2319) -> (40.2184, 14.5248) projected
  line L291 (40.2184, 14.5248) -> (40.9255, 15.2319) projected
  line L292 (40.9255, 15.2319) -> (40.2184, 15.939) projected
  line L293 (40.2184, 15.939) -> (40.9255, 16.6461) projected
  line L294 (40.9255, 16.6461) -> (41.6326, 15.939) projected
  line L295 (41.6326, 15.939) -> (42.3397, 16.6461) projected
  line L296 (42.3397, 16.6461) -> (41.6326, 17.3532) projected
  line L297 (41.6326, 17.3532) -> (42.3397, 18.0603) projected
  line L298 (42.3397, 18.0603) -> (43.0468, 17.3532) projected
  line L299 (43.0468, 17.3532) -> (43.7539, 18.0603) projected
  line L300 (43.7539, 18.0603) -> (43.0468, 18.7674) projected
  line L301 (43.0468, 18.7674) -> (43.7539, 19.4745) projected
  line L302 (43.7539, 19.4745) -> (44.461, 18.7674) projected
  line L303 (44.461, 18.7674) -> (45.1681, 19.4745) projected
  line L304 (45.1681, 19.4745) -> (45.1681, 21.7092) projected
  line L305 (45.1681, 21.7092) -> (44.1681, 21.7092) projected
  line L306 (44.1681, 21.7092) -> (44.1681, 22.7092) projected
  line L307 (44.1681, 22.7092) -> (45.1681, 22.7092) projected
  line L308 (45.1681, 22.7092) -> (45.1681, 23.7092) projected
  line L309 (45.1681, 23.7092) -> (44.1681, 23.7092) projected
  line L310 (44.1681, 23.7092) -> (44.1681, 24.7092) projected
  line L311 (44.1681, 24.7092) -> (45.1681, 24.7092) projected
  line L312 (45.1681, 24.7092) -> (45.1681, 25.7092) projected
  line L313 (45.1681, 25.7092) -> (44.1681, 25.7092) projected
  line L314 (44.1681, 25.7092) -> (44.1681, 26.7092) projected
  line L315 (44.1681, 26.7092) -> (45.1681, 26.7092) projected
  line L316 (45.1681, 26.7092) -> (45.1681, 27.7092) projected
  line L317 (45.1681, 27.7092) -> (44.1681, 27.7092) projected
  line L318 (44.1681, 27.7092) -> (44.1681, 28.7092) projected
  line L319 (44.1681, 28.7092) -> (45.1681, 28.7092) projected
  line L320 (45.1681, 28.7092) -> (45.1681, 29.7092) projected
  line L321 (45.1681, 29.7092) -> (44.1681, 29.7092) projected
  line L322 (44.1681, 29.7092) -> (44.1681, 30.7092) projected
  line L323 (44.1681, 30.7092) -> (45.1681, 30.7092) projected
  line L324 (45.1681, 30.7092) -> (45.1681, 31.7092) projected
  line L325 (45.1681, 31.7092) -> (44.1681, 31.7092) projected
  line L326 (44.1681, 31.7092) -> (44.1681, 32.7092) projected
  line L327 (44.1681, 32.7092) -> (45.1681, 32.7092) projected
  line L328 (45.1681, 32.7092) -> (45.1681, 33.7092) projected
  line L329 (45.1681, 33.7092) -> (44.1681, 33.7092) projected
  line L330 (44.1681, 33.7092) -> (44.1681, 34.7092) projected
  line L331 (44.1681, 34.7092) -> (45.1681, 34.7092) projected
  line L332 (45.1681, 34.7092) -> (45.1681, 35.7092) projected
  line L333 (45.1681, 35.7092) -> (44.1681, 35.7092) projected
  line L334 (44.1681, 35.7092) -> (44.1681, 36.7092) projected
  line L335 (44.1681, 36.7092) -> (45.1681, 36.7092) projected
  line L336 (45.1681, 36.7092) -> (45.1681, 37.7092) projected
  line L337 (45.1681, 37.7092) -> (44.1681, 37.7092) projected
  line L338 (44.1681, 37.7092) -> (44.1681, 38.7092) projected
  line L339 (44.1681, 38.7092) -> (45.1681, 38.7092) projected
  line L340 (45.1681, 38.7092) -> (45.1681, 39.7092) projected
  line L341 (45.1681, 39.7092) -> (44.1681, 39.7092) projected
  line L342 (44.1681, 39.7092) -> (44.1681, 40.7092) projected
  line L343 (44.1681, 40.7092) -> (45.1681, 40.7092) projected
  line L344 (45.1681, 40.7092) -> (45.1681, 41.7092) projected
  line L345 (45.1681, 41.7092) -> (44.1681, 41.7092) projected
  line L346 (44.1681, 41.7092) -> (44.1681, 42.7092) projected
  line L347 (44.1681, 42.7092) -> (45.1681, 42.7092) projected
  line L348 (45.1681, 42.7092) -> (45.1681, 43.7092) projected
  line L349 (45.1681, 43.7092) -> (44.1681, 43.7092) projected
  line L350 (44.1681, 43.7092) -> (44.1681, 44.7092) projected
  line L351 (44.1681, 44.7092) -> (45.1681, 44.7092) projected
  line L352 (45.1681, 44.7092) -> (45.1681, 45.7092) projected
  line L353 (45.1681, 45.7092) -> (43.5879, 47.2894) projected
  line L354 (43.5879, 47.2894) -> (42.8808, 46.5823) projected
  line L355 (42.8808, 46.5823) -> (42.1737, 47.2894) projected
  line L356 (42.1737, 47.2894) -> (42.8808, 47.9965) projected
  line L357 (42.8808, 47.9965) -> (42.1737, 48.7037) projected
  line L358 (42.1737, 48.7037) -> (41.4666, 47.9965) projected
  line L359 (41.4666, 47.9965) -> (40.7595, 48.7037) projected
  line L360 (40.7595, 48.7037) -> (41.4666, 49.4108) projected
  line L361 (41.4666, 49.4108) -> (40.7595, 50.1179) projected
  line L362 (40.7595, 50.1179) -> (40.0524, 49.4108) projected
  line L363 (40.0524, 49.4108) -> (39.3453, 50.1179) projected
  line L364 (39.3453, 50.1179) -> (40.0524, 50.825) projected
  line L365 (40.0524, 50.825) -> (39.3453, 51.5321) projected
  line L366 (39.3453, 51.5321) -> (38.6382, 50.825) projected
  line L367 (38.6382, 50.825) -> (37.9311, 51.5321) projected
  line L368 (37.9311, 51.5321) -> (38.6382, 52.2392) projected
  line L369 (38.6382, 52.2392) -> (37.9311, 52.9463) projected
  line L370 (37.9311, 52.9463) -> (37.224, 52.2392) projected
  line L371 (37.224, 52.2392) -> (36.5169, 52.9463) projected
  line L372 (36.5169, 52.9463) -> (37.224, 53.6534) projected
  line L373 (37.224, 53.6534) -> (36.5169, 54.3605) projected
  line L374 (36.5169, 54.3605) -> (35.8098, 53.6534) projected
  line L375 (35.8098, 53.6534) -> (35.1026, 54.3605) projected
  line L376 (35.1026, 54.3605) -> (35.8098, 55.0676) projected
  line L377 (35.8098, 55.0676) -> (35.1026, 55.7747) projected
  line L378 (35.1026, 55.7747) -> (34.3955, 55.0676) projected
  line L379 (34.3955, 55.0676) -> (33.6884, 55.7747) projected
  line L380 (33.6884, 55.7747) -> (34.3955, 56.4818) projected
  line L381 (34.3955, 56.4818) -> (33.6884, 57.1889) projected
  line L382 (33.6884, 57.1889) -> (32.9813, 56.4818) projected
  line L383 (32.9813, 56.4818) -> (32.2742, 57.1889) projected
  line L384 (32.2742, 57.1889) -> (32.9813, 57.896) projected
  line L385 (32.9813, 57.896) -> (32.2742, 58.6032) projected
  line L386 (32.2742, 58.6032) -> (31.5671, 57.896) projected
  line L387 (31.5671, 57.896) -> (30.86, 58.6032) projected
  line L388 (30.86, 58.6032) -> (31.5671, 59.3103) projected
  line L389 (31.5671, 59.3103) -> (30.86, 60.0174) projected
  line L390 (30.86, 60.0174) -> (30.1529, 59.3103) projected
  line L391 (30.1529, 59.3103) -> (29.4458, 60.0174) projected
  line L392 (37.6421, 22.5919) -> (23.5, 8.4497) projected
  line L393 (23.5, 8.4497) -> (3.5, 8.4497) projected
  line L394 (3.5, 8.4497) -> (-10.6421, 22.5919) projected
  line L395 (-10.6421, 22.5919) -> (-10.6421, 42.5919) projected
  line L396 (-10.6421, 42.5919) -> (3.5, 56.734) projected
  line L397 (3.5, 56.734) -> (23.5, 56.734) projected
  line L398 (23.5, 56.734) -> (37.6421, 42.5919) projected
  line L399 (37.6421, 42.5919) -> (37.6421, 22.5919) projected
extrude "돌출2" add sketch "스케치2" along normal blind 5 contours L392 L393 L394 L395 L396 L397 L398 L399
ref_plane "작업 평면1" through (-13.4999, 0, 82.7525) normal (-1, 0, 0) x (0, 0, -1)